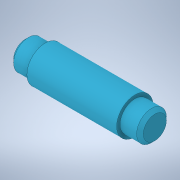
# Autodesk Inventor part: axle
Saved by Autodesk Inventor 2020 (Build 240168000, 168)
## iProperties
Created: 2021-06-13
Part Number: axle
Material: Stainless Steel
Document SubType Name: Modeling
Designer: joelm
Density: 8 g/cm^3
Appearance: Turquoise
Mass: 209.379 g
Surface Area: 56.7607 cm^2
Volume: 26.1724 cm^3
Author: joelm
Autodesk Inventor part; units mm, degrees
ref_plane "YZ Plane" through (0, 0, 0) normal (1, 0, 0) x (0, 1, 0)
ref_plane "XZ Plane" through (0, 0, 0) normal (0, 1, 0) x (-1, 0, 0)
ref_plane "XY Plane" through (0, 0, 0) normal (0, 0, 1) x (1, 0, 0)
sketch "Sketch1" plane through (0, 0, 0) normal (0, 0, 1) x (1, 0, 0)
  line L0 (0, 0) -> (78, 0)
  line L1 (78, 0) -> (78, 8.95)
  line L2 (78, 8.95) -> (66, 8.95)
  line L3 (66, 8.95) -> (66, 10.95)
  line L4 (66, 10.95) -> (12, 10.95)
  line L5 (12, 10.95) -> (12, 8.95)
  line L6 (12, 8.95) -> (0, 8.95)
  line L7 (0, 8.95) -> (0, 0)
  dimension "d0" = 78
  dimension "d1" = 8.95
  dimension "d2" = 12
  dimension "d3" = 2
  dimension "d4" = 54
  dimension "d5" = 2
  constraints: 16 end point, 5 perpendicular, 2 point on line, 1 horizontal
  measures "d0" distance of L0.start L0.end
  measures "d1" distance of L0.end L1.end
  measures "d2" distance of L1.end L2.end
  measures "d3" distance of L2.end L3.end
  measures "d4" distance of L3.end L4.end
  measures "d5" distance of L4.end L5.end
revolve "Revolution1" add sketch "Sketch1" angle 360 about axis through (0, 0, 0) along (1, 0, 0)
chamfer "Chamfer1" distance 2 angle 45 1 edges at (78, -8.95, 0) measured on face at (78, -8.45, 0)
chamfer "Chamfer2" distance 2 angle 45 1 edges at (0, -8.95, 0) measured on face at (0, -8.45, 0)
body "Solid1"
